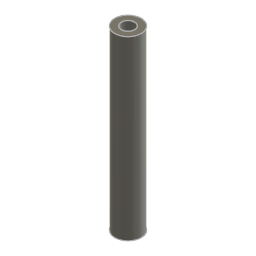
barras 40mm (Autodesk Fusion 360 design; units mm, degrees)
part number: 2026-06-22-23-55-10-797
Autodesk Fusion 360 part; units mm, degrees
sketch "Boceto1" plane through (0, 0, 0) normal (0, 1, 0) x (1, 0, 0)
  circle A0 centre (0, 0) radius 3
  dimension "d1" = 6
  constraint coincident A0.centre origin
  measures "d1" diameter of A0
extrude "Extruir1" add sketch "Boceto1" along normal blind 40
sketch "Boceto2" plane through (0, 40, 0) normal (0, 1, 0) x (-1, 0, 0)
  circle A0 centre (0, 0) radius 3
  circle A1 centre (0, 0) radius 1.525
  dimension "d4" = 3.05
  constraint coincident A0.centre A1.centre
  measures "d4" diameter of A1
sketch "Boceto3" plane through (0, 0, 0) normal (0, -1, 0) x (1, 0, 0)
  circle A0 centre (0, 0) radius 3
  circle A1 centre (0, 0) radius 1.525
  dimension "d5" = 3.05
  constraint concentric A0 A1
  measures "d5" diameter of A1
hole "Agujero1" at (0, 40, 0) direction (0, -1, 0) diameter 3 depth 10 tip angle 118
hole "Agujero2" at (0, 0, 0) direction (0, 1, 0) diameter 3 depth 10 tip angle 118
